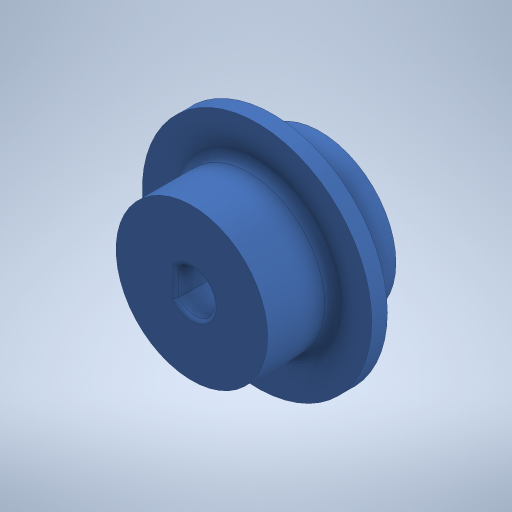
# Autodesk Inventor part: Knob_adp
Saved by Autodesk Inventor 2024 (Build 280153000, 153)
## iProperties
Created: 2022-02-14
Part Number: Knob_adp
Material: Generic
Document SubType Name: Modeling
Designer: la8011
Density: 1 g/cm^3
Appearance: Default(1)
Author: la8011
Autodesk Inventor part; units mm, degrees
ref_plane "YZ Plane" through (0, 0, 0) normal (1, 0, 0) x (0, 1, 0)
ref_plane "XZ Plane" through (0, 0, 0) normal (0, 1, 0) x (-1, 0, 0)
ref_plane "XY Plane" through (0, 0, 0) normal (0, 0, 1) x (1, 0, 0)
sketch "Sketch1" plane through (0, 0, 0) normal (0, 1, 0) x (-1, 0, 0)
  line L0 (0, 0) -> (2, 0)
  line L1 (2, 0) -> (2, 8.15)
  line L2 (2, 8.15) -> (0, 8.15)
  line L3 (0, 8.15) -> (0, 0)
  line L4 (0, 8.15) -> (9.25, 8.15)
  line L5 (9.25, 8.15) -> (9.25, 15.65)
  line L6 (9.25, 15.65) -> (0, 15.65)
  line L7 (0, 15.65) -> (0, 8.15)
  line L8 (0, 7.7) -> (-4.75, 7.7)
  line L9 (-4.75, 7.7) -> (-4.75, 5.8)
  line L10 (-4.75, 5.8) -> (0, 5.8)
  line L11 (0, 5.8) -> (0, 7.7)
  point P0 (0, 5.8)
  dimension "d1" = 7.25
  dimension "d2" = 2
  dimension "d3" = 7.5
  dimension "d4" = 8.15
  dimension "d10" = 14
  dimension "d12" = 1.9
  dimension "d13" = 7.95
  constraints: 24 end point, 6 parallel, 3 horizontal, 3 perpendicular, 1 point on line
  measures "d1" distance between parallel lines of L1 L5
  measures "d2" distance between parallel lines of L7 L1
  measures "d3" distance between parallel lines of L6 L4
  measures "d4" distance between parallel lines of L0 L4
  measures "d10" distance between parallel lines of L5 L9
  measures "d12" distance between parallel lines of L8 L10
  measures "d13" distance between parallel lines of L6 L8
revolve "Revolution1" add sketch "Sketch1" angle 360 about axis through (-9.25, 0, 8.15) along (0, 0, 1)
sketch "Sketch2" plane through (-9.25, 0, 15.65) normal (0, 0, 1) x (1, 0, 0)
  circle A0 centre (0, 0) radius 2.6
  line L0 (-2.0092, 1.6502) -> (-1.9908, -1.6724)
  circle A1 centre (0, 0) radius 9.25 projected
  circle A2 centre (0, 0) radius 9.4
  point P0 (9.25, 0)
  dimension "d6" = 5.2
  dimension "d7" = 2
  constraints: 2 centre point, 2 end point, 2 point on circle, 1 coincident, 1 horizontal alignment, 1 other
  measures "d6" diameter of A0
  measures "d7" distance from line of L0 A0.centre
extrude "Extrusion1" cut sketch "Sketch2" against normal blind 10 contours A0 L0 picked at (-0.3829, 0.5768)
fillet "Fillet1" radius 1 2 edges at (-18.5, 0, 7.7) (-18.5, 0, 5.8)
fillet "Fillet2" radius 0.4 2 edges at (-6.65, 0.0144, 15.65) (-11.25, -0.0111, 15.65)
body "Solid1"
